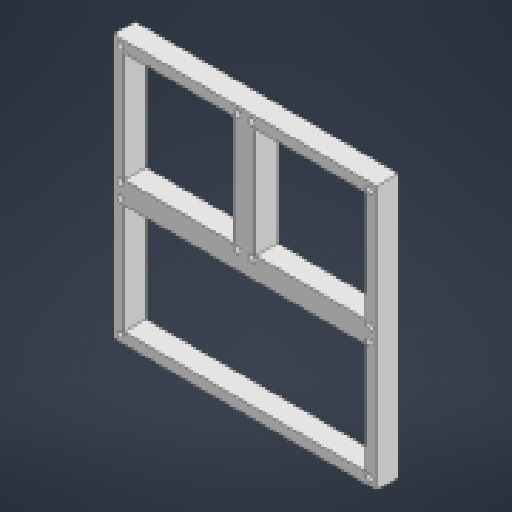
# Autodesk Inventor part: frame_demo_2x2_xyxx
Saved by Autodesk Inventor 2024 (Build 280153000, 153)
## iProperties
Created: 2026-05-08
Part Number: frame_demo_2x2_xyxx
Material: Generic
Document SubType Name: Modeling
Designer: schar
Density: 1 g/cm^3
Appearance: Default
Author: schar
Autodesk Inventor part; units mm, degrees
ref_plane "YZ Plane" through (0, 0, 0) normal (1, 0, 0) x (0, 1, 0)
ref_plane "XZ Plane" through (0, 0, 0) normal (0, 1, 0) x (-1, 0, 0)
ref_plane "XY Plane" through (0, 0, 0) normal (0, 0, 1) x (1, 0, 0)
sketch "Sketch1" plane through (0, 0, 0) normal (0, 0, 1) x (1, 0, 0)
  line L0 (-79, -35) -> (19, -35) projected
  line L1 (25, -41) -> (25, -79) projected
  line L2 (30, -32) -> (30, -36) projected
  line L3 (30, -24) -> (30, -28) projected
  line L4 (28, -30) -> (24, -30) projected
  line L5 (-24, -30) -> (-28, -30) projected
  line L6 (-30, -28) -> (-30, -24) projected
  line L7 (-88, -30) -> (-84, -30) projected
  line L8 (-85, -79) -> (-85, -41) projected
  line L9 (19, -85) -> (-79, -85) projected
  line L10 (30, -84) -> (30, -88) projected
  line L11 (24, -90) -> (19, -85) projected
  line L12 (28, -90) -> (24, -90) projected
  line L13 (-84, -90) -> (-88, -90) projected
  line L14 (-90, -88) -> (-90, -84) projected
  line L15 (-30, 24) -> (-30, 28) projected
  line L16 (-28, 30) -> (-24, 30) projected
  line L17 (24, 30) -> (28, 30) projected
  line L18 (30, 28) -> (30, 24) projected
  line L19 (25, 19) -> (25, -19) projected
  line L20 (-25, -19) -> (-25, 19) projected
  line L21 (19, -25) -> (-19, -25) projected
  line L22 (-19, 25) -> (19, 25) projected
  line L23 (25, 25) -> (-25, 25)
  line L24 (-25, 25) -> (-25, -25)
  line L25 (-25, -25) -> (25, -25)
  line L26 (25, -25) -> (25, 25)
  line L27 (25, -35) -> (-85, -35)
  line L28 (-85, -35) -> (-85, -85)
  line L29 (-85, -85) -> (25, -85)
  line L30 (25, -85) -> (25, -35)
  line L31 (30, -30) -> (-90, -30)
  line L32 (-90, -30) -> (-90, -90)
  line L33 (-90, -90) -> (30, -90)
  line L34 (30, -90) -> (30, -30)
  line L35 (30, 30) -> (-30, 30)
  line L36 (-30, 30) -> (-30, -30)
  line L37 (-30, -30) -> (30, -30)
  line L38 (30, -30) -> (30, 30)
  line L39 (-30, -30) -> (-90, -30)
  line L40 (-90, -30) -> (-90, 30)
  line L41 (-90, 30) -> (-30, 30)
  line L42 (-30, 30) -> (-30, -30)
  line L43 (-30, -25) -> (-35, -25)
  line L44 (-35, -25) -> (-85, -25)
  line L45 (-85, -25) -> (-85, 25)
  line L46 (-85, 25) -> (-35, 25)
  line L47 (-35, 25) -> (-35, -25)
  circle A0 centre (-26.7678, 26.7678) radius 1.5 projected
  circle A1 centre (26.7678, 26.7678) radius 1.5 projected
  circle A2 centre (26.7678, -26.7678) radius 1.5 projected
  circle A3 centre (-26.7678, -26.7678) radius 1.5 projected
  circle A4 centre (26.768, -33.232) radius 1.5 projected
  circle A5 centre (26.768, -86.768) radius 1.5 projected
  circle A6 centre (-86.768, -86.768) radius 1.5 projected
  circle A7 centre (-86.768, -33.232) radius 1.5 projected
  circle A8 centre (-33.2322, 26.7678) radius 1.5
  circle A9 centre (-86.7678, 26.7678) radius 1.5
  circle A10 centre (-86.7678, -26.7678) radius 1.5
  circle A11 centre (-33.2322, -26.7678) radius 1.5
  point P0 (0, 0)
  dimension "d0" = 5
  constraints: 50 end point, 12 parallel, 7 perpendicular, 6 horizontal, 5 point on line, 4 centre point, 4 symmetric about line, 1 midpoint, 4 other
  measures "d0" distance of L43.start L43.end
extrude "Extrusion1" add sketch "Sketch1" along normal blind 10
fillet "Fillet1" radius 2 4 edges at (-90, 30, 5) (-90, -90, 5) (30, -90, 5) (30, 30, 5)
body "Solid1"
